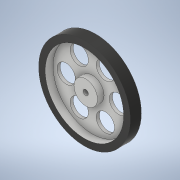
# Autodesk Inventor part: 70アルミホイール内径６ (1)
Saved by Autodesk Inventor 2020 (Build 240168000, 168)
## iProperties
Created: 2021-05-15
Part Number: 70アルミホイール内径６ (1)
Material: 一般
Document SubType Name: Modeling
Designer: fmasa
Density: 2.0963 g/cm^3
Appearance: 既定
Mass: 30 g
Surface Area: 98.6774 cm^2
Volume: 14.3109 cm^3
Author: fmasa
Autodesk Inventor part; units mm, degrees
ref_plane "YZ Plane" through (0, 0, 0) normal (1, 0, 0) x (0, 1, 0)
ref_plane "XZ Plane" through (0, 0, 0) normal (0, 1, 0) x (-1, 0, 0)
ref_plane "XY Plane" through (0, 0, 0) normal (0, 0, 1) x (1, 0, 0)
sketch "スケッチ1" plane through (0, 0, 0) normal (0, 0, 1) x (1, 0, 0)
  circle A0 centre (0, 0) radius 35
  dimension "d0" = 70
  constraints: 1 centre point, 1 coincident
  measures "d0" diameter of A0
extrude "押し出し1" add sketch "スケッチ1" along normal blind 8.5
sketch "スケッチ2" plane through (0, 0, 8.5) normal (0, 0, 1) x (1, 0, 0)
  circle A0 centre (0, 0) radius 35 projected
  circle A1 centre (0, 0) radius 30
  dimension "d3" = 5
  constraints: 1 centre point
  measures "d3" radial gap between concentric circles of A0 A1
extrude "押し出し2" cut sketch "スケッチ2" against normal blind 6 contours A1
sketch "スケッチ3" plane through (0, 0, 2.5) normal (0, 0, 1) x (1, 0, 0)
  circle A0 centre (0, 0) radius 2
  circle A1 centre (0, 0) radius 9
  dimension "d7" = 4
  dimension "d8" = 18
  constraints: 2 centre point, 2 coincident
  measures "d7" diameter of A0
  measures "d8" diameter of A1
extrude "押し出し3" add sketch "スケッチ3" along normal blind 5
extrude "押し出し4" cut sketch "スケッチ3" against normal blind 5 contours A0
sketch "スケッチ4" plane through (0, 0, 2.5) normal (0, 0, 1) x (1, 0, 0)
  circle A0 centre (20, 0) radius 7
  circle A1 centre (10, 17.3205) radius 7
  circle A2 centre (-10, 17.3205) radius 7
  circle A3 centre (-20, 0) radius 7
  circle A4 centre (-10, -17.3205) radius 7
  circle A5 centre (10, -17.3205) radius 7
  point P0 (0, 0)
  dimension "d14" = 14
  dimension "d15" = 20
  dimension "d18" = 360
  constraints: 6 centre point, 13 other
  measures "d14" diameter of A0
  measures "d15" distance of A0.centre point (0, 0)
extrude "押し出し5" cut sketch "スケッチ4" against normal blind 5
sketch "スケッチ5" plane through (0, 0, 0) normal (0, 0, -1) x (-1, 0, 0)
  circle A0 centre (0, 0) radius 2 projected
  circle A1 centre (0, 0) radius 30
  constraints: 1 centre point, 1 coincident
extrude "押し出し6" cut sketch "スケッチ5" against normal blind 0.1
